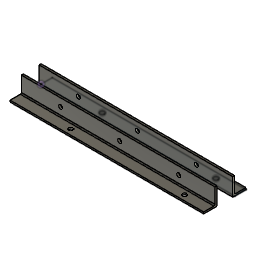
24v mount v1 (Autodesk Fusion 360 design; units mm, degrees)
Autodesk Fusion 360 part; units mm, degrees
sketch "Sketch1" plane through (0, 0, 0) normal (0, 0, 1) x (1, 0, 0)
  line L0 (0, 0) -> (196.85, 0)
  line L1 (196.85, 0) -> (196.85, 11.46)
  line L2 (196.85, 11.46) -> (0, 11.46)
  line L3 (0, 11.46) -> (0, 0)
  circle A0 centre (56.28, 5.96) radius 2.2
  circle A1 centre (171.87, 5.96) radius 2.2
  dimension "d1" = 196.85
  dimension "d2" = 11.46
  dimension "d5" = 4.4
  dimension "d6" = 56.28
  dimension "d7" = 4.4
  dimension "d8" = 24.98
  dimension "d9" = 5.5
  dimension "d10" = 5.5
  constraint horizontal L0
  constraint vertical L1
  constraint horizontal L2
  constraint vertical L3
  constraint coincident L0.start L3.end
  measures "d1" distance of L0.start L0.end
  measures "d2" distance of L0 L2
  measures "d5" diameter of A0
  measures "d6" distance of L3 A0.centre
  measures "d7" diameter of A1
  measures "d8" distance of L1 A1.centre
  measures "d9" distance of L2 A0.centre
  measures "d10" distance of L2 A1.centre
extrude "Extrude1" add sketch "Sketch1" along normal blind 1.65 contours L0 L1 L2 L3 | A0 | A1 makes body 1
extrude "Extrude2" cut sketch "Sketch1" along normal through all contours A0 | A1 bodies 1
sketch "Sketch2" plane through (0, 0, 0) normal (0, 1, 0) x (1, 0, 0)
  line L0 (0, 0) -> (196.85, 0)
  line L1 (196.85, 0) -> (196.85, -18)
  line L2 (196.85, -18) -> (0, -18)
  line L3 (0, -18) -> (0, 0)
  dimension "d12" = 196.85
  dimension "d13" = 18
  constraint horizontal L0
  constraint vertical L1
  constraint horizontal L2
  constraint vertical L3
  constraint coincident L0.start L3.end
  measures "d12" distance of L0.start L0.end
  measures "d13" distance of L0.start L2.end
extrude "Extrude3" add sketch "Sketch2" against normal blind 2 bodies 1
fillet "Fillet1" radius 1 1 edges at (98.425, 0, 1.65) on bodies 1
sketch "Sketch3" plane through (0, 0, 0) normal (0, 1, 0) x (-1, 0, 0)
  line L0 (-196.85, 2.65) -> (0, 2.65)
  line L1 (0, 2.65) -> (0, 18)
  line L2 (0, 18) -> (-196.85, 18)
  line L3 (-196.85, 18) -> (-196.85, 2.65)
  circle A0 centre (-160, 10) radius 2
  circle A1 centre (-100, 10) radius 2
  circle A2 centre (-40, 10) radius 2
  dimension "d18" = 4
  dimension "d19" = 4
  dimension "d20" = 4
  measures "d18" diameter of A0
  measures "d19" diameter of A1
  measures "d20" diameter of A2
extrude "Extrude4" cut sketch "Sketch3" against normal blind 5 contours A0 | A1 | A2 bodies 1
ref_plane "WorkPlane1" through (0, -10, 0) normal (0, 1, 0) x (0, 0, 1)
mirror "Mirror1" about plane through (0, -10, 0) normal (0, 1, 0) of bodies 1 makes body 2
